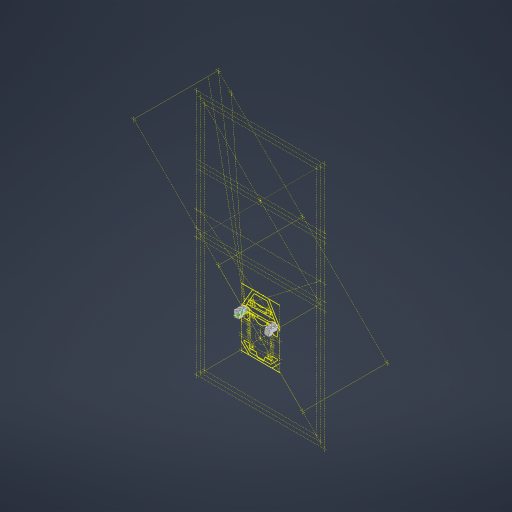
# Autodesk Inventor part: sensormount-2
Saved by Autodesk Inventor 2023.5 (Build 275446000, 446)
## iProperties
Created: 2025-01-19
Part Number: sensormount-2
Material: 一般
Document SubType Name: Modeling
Designer: IshiiLabHonda
Density: 1 g/cm^3
Appearance: 既定
Author: IshiiLabHonda
Autodesk Inventor part; units mm, degrees
ref_plane "YZ Plane" through (0, 0, 0) normal (1, 0, 0) x (0, 1, 0)
ref_plane "XZ Plane" through (0, 0, 0) normal (0, 1, 0) x (-1, 0, 0)
ref_plane "XY Plane" through (0, 0, 0) normal (0, 0, 1) x (1, 0, 0)
derived "chassis.ipt"
sketch "スケッチ1" plane through (0, 0, 0) normal (0, 0, 1) x (1, 0, 0)
  line L0 (-90, 90) -> (90, 90) construction
  line L1 (90, 90) -> (90, -90) construction
  line L2 (90, -90) -> (-90, -90) construction
  line L3 (-90, -90) -> (-90, 90) construction
  line L4 (-90, 90) -> (-90, 270) construction
  line L5 (-90, 270) -> (90, 270) construction
  line L6 (90, 270) -> (90, 90) construction
  line L7 (-90, 90) -> (90, -90) construction
  line L8 (90, 90) -> (-90, -90) construction
  line L9 (0, 0) -> (0, 10) construction
  line L10 (0, 0) -> (10, 0) construction
  line L11 (-90, 270) -> (90, 90) construction
  line L12 (-90, 90) -> (90, 270) construction
  line L13 (-96, 276) -> (96, 276) construction
  line L14 (96, 276) -> (96, -96) construction
  line L15 (96, -96) -> (-96, -96) construction
  line L16 (-96, -96) -> (-96, 276) construction
  line L17 (-84, 264) -> (84, 264) construction
  line L18 (84, 264) -> (84, -84) construction
  line L19 (84, -84) -> (-84, -84) construction
  line L20 (-84, -84) -> (-84, 264) construction
  line L21 (-96, 96) -> (96, 96) construction
  line L22 (-96, 84) -> (96, 84) construction
  line L23 (-63.6396, 63.6396) -> (63.6396, 190.9188) construction
  line L24 (63.6396, 190.9188) -> (190.9188, 63.6396) construction
  line L25 (190.9188, 63.6396) -> (63.6396, -63.6396) construction
  line L26 (63.6396, -63.6396) -> (-63.6396, 63.6396) construction
  line L27 (-190.9188, 190.9188) -> (-63.6396, 318.1981) construction
  line L28 (-63.6396, 318.1981) -> (63.6396, 190.9188) construction
  line L29 (-63.6396, 63.6396) -> (-190.9188, 190.9188) construction
  line L30 (-96, 120) -> (96, 120) construction
  line L31 (-96, 186) -> (96, 186) construction
  line L32 (-96, 174) -> (96, 174) construction
  line L33 (-96, 180) -> (96, 180) construction
  point P0 (-63.6396, 318.1981)
  point P1 (-90, 120)
  point P2 (90, 120)
  point P3 (0, 180)
sketch "スケッチ2" plane through (0, 0, 0) normal (0, 0, 1) x (1, 0, 0)
  line L0 (63.6396, 190.9188) -> (190.9188, 63.6396) construction
  line L1 (-63.6396, 318.1981) -> (63.6396, 190.9188) construction
  line L2 (-84, 264) -> (84, 264) construction
  line L3 (-90, 270) -> (90, 270) construction
  line L4 (90, 270) -> (90, 90) construction
  line L5 (-96, 276) -> (96, 276) construction
  line L6 (-90, 90) -> (90, 270) construction
  line L7 (-90, 270) -> (90, 90) construction
  line L8 (-63.6396, 63.6396) -> (63.6396, 190.9188) construction
  line L9 (-96, 120) -> (96, 120) construction
  line L10 (-90, 90) -> (90, 90) construction
  line L11 (-96, 96) -> (96, 96) construction
  line L12 (-96, 84) -> (96, 84) construction
  line L13 (90, -90) -> (-90, -90) construction
  line L14 (0, 0) -> (0, 10) construction
  line L15 (0, 0) -> (10, 0) construction
  line L16 (190.9188, 63.6396) -> (63.6396, -63.6396) construction
  line L17 (63.6396, -63.6396) -> (-63.6396, 63.6396) construction
  line L18 (84, -84) -> (-84, -84) construction
  line L19 (96, -96) -> (-96, -96) construction
  line L20 (-90, 90) -> (-90, 270) construction
  line L21 (-63.6396, 63.6396) -> (-190.9188, 190.9188) construction
  line L22 (-190.9188, 190.9188) -> (-63.6396, 318.1981) construction
  line L23 (96, 276) -> (96, -96) construction
  line L24 (-96, -96) -> (-96, 276) construction
  line L25 (84, 264) -> (84, -84) construction
  line L26 (-84, -84) -> (-84, 264) construction
  line L27 (90, 90) -> (90, -90) construction
  line L28 (-90, 90) -> (90, -90) construction
  line L29 (90, 90) -> (-90, -90) construction
  line L30 (-90, -90) -> (-90, 90) construction
  circle A0 centre (0, 0) radius 16 construction
  circle A1 centre (0, 0) radius 7.5 construction
  line L31 (20, 11.5) -> (28.75, 11.5) construction
  line L32 (28.75, 11.5) -> (28.75, -11.5) construction
  line L33 (28.75, -11.5) -> (20, -11.5) construction
  line L34 (20, -11.5) -> (20, 11.5) construction
  line L35 (20, 11.5) -> (18, 11.5) construction
  line L36 (18, 11.5) -> (18, -11.5) construction
  line L37 (18, -11.5) -> (20, -11.5) construction
  line L38 (18, 1.5) -> (17, 1.5) construction
  line L39 (17, -1.5) -> (18, -1.5) construction
  line L40 (-17, 26) -> (17, 26) construction
  line L41 (17, 26) -> (17, -20) construction
  line L42 (17, -20) -> (-17, -20) construction
  line L43 (-17, -20) -> (-17, 26) construction
  line L44 (-20, 11.5) -> (-18, 11.5) construction
  line L45 (-17, -1.5) -> (-18, -1.5) construction
  line L46 (-20, -11.5) -> (-20, 11.5) construction
  line L47 (-18, 11.5) -> (-18, -11.5) construction
  line L48 (-28.75, -11.5) -> (-20, -11.5) construction
  line L49 (-20, 11.5) -> (-28.75, 11.5) construction
  line L50 (-28.75, 11.5) -> (-28.75, -11.5) construction
  line L51 (-18, -11.5) -> (-20, -11.5) construction
  line L52 (-18, 1.5) -> (-17, 1.5) construction
  line L53 (-14.5, 26) -> (-14.5, -20) construction
  line L54 (14.5, 26) -> (14.5, -20) construction
  line L55 (-10.5, 26) -> (-10.5, 21) construction
  line L56 (-10.5, 21) -> (-14.5, 21) construction
  line L57 (-14.5, 26) -> (-10.5, 21) construction
  line L58 (-10.5, 26) -> (-14.5, 21) construction
  circle A2 centre (-12.5, 23.5) radius 1 construction
  line L59 (10.5, 26) -> (10.5, 21) construction
  line L60 (10.5, 21) -> (14.5, 21) construction
  line L61 (10.5, 26) -> (14.5, 21) construction
  line L62 (10.5, 21) -> (14.5, 26) construction
  circle A3 centre (12.5, 23.5) radius 1 construction
  line L63 (-14.5, -15) -> (-10.5, -15) construction
  line L64 (-10.5, -15) -> (-10.5, -20) construction
  line L65 (10.5, -20) -> (10.5, -15) construction
  line L66 (10.5, -15) -> (14.5, -15) construction
  line L67 (-14.5, -15) -> (-10.5, -20) construction
  line L68 (-10.5, -15) -> (-14.5, -20) construction
  circle A4 centre (-12.5, -17.5) radius 1 construction
  line L69 (10.5, -15) -> (14.5, -20) construction
  line L70 (14.5, -15) -> (10.5, -20) construction
  circle A5 centre (12.5, -17.5) radius 1 construction
  point P0 (90, 120)
  point P1 (-90, 120)
  point P2 (-63.6396, 318.1981)
  point P3 (-12.5, -17.5)
sketch "スケッチ3" plane through (0, 0, 0) normal (0, 0, 1) x (1, 0, 0)
  line L0 (63.6396, 190.9188) -> (190.9188, 63.6396) construction
  line L1 (-63.6396, 318.1981) -> (63.6396, 190.9188) construction
  line L2 (-84, 264) -> (84, 264) construction
  line L3 (-90, 270) -> (90, 270) construction
  line L4 (90, 270) -> (90, 90) construction
  line L5 (-96, 276) -> (96, 276) construction
  line L6 (-90, 90) -> (90, 270) construction
  line L7 (-90, 270) -> (90, 90) construction
  line L8 (-63.6396, 63.6396) -> (63.6396, 190.9188) construction
  line L9 (-96, 120) -> (96, 120) construction
  line L10 (-90, 90) -> (90, 90) construction
  line L11 (-96, 96) -> (96, 96) construction
  line L12 (-96, 84) -> (96, 84) construction
  line L13 (90, -90) -> (-90, -90) construction
  line L14 (0, 0) -> (0, 10) construction
  line L15 (0, 0) -> (10, 0) construction
  line L16 (190.9188, 63.6396) -> (63.6396, -63.6396) construction
  line L17 (63.6396, -63.6396) -> (-63.6396, 63.6396) construction
  line L18 (84, -84) -> (-84, -84) construction
  line L19 (96, -96) -> (-96, -96) construction
  line L20 (-90, 90) -> (-90, 270) construction
  line L21 (-63.6396, 63.6396) -> (-190.9188, 190.9188) construction
  line L22 (-190.9188, 190.9188) -> (-63.6396, 318.1981) construction
  line L23 (96, 276) -> (96, -96) construction
  line L24 (-96, -96) -> (-96, 276) construction
  line L25 (84, 264) -> (84, -84) construction
  line L26 (-84, -84) -> (-84, 264) construction
  line L27 (90, 90) -> (90, -90) construction
  line L28 (-90, 90) -> (90, -90) construction
  line L29 (90, 90) -> (-90, -90) construction
  line L30 (-90, -90) -> (-90, 90) construction
  line L31 (-18, 1.5) -> (-17, 1.5) construction
  line L32 (-17, -1.5) -> (-18, -1.5) construction
  line L33 (-20, 11.5) -> (-18, 11.5) construction
  line L34 (-28.75, 11.5) -> (-28.75, -11.5) construction
  line L35 (63.6396, -63.6396) -> (-63.6396, 63.6396) construction
  line L36 (84, -84) -> (-84, -84) construction
  line L37 (-90, -90) -> (-90, 90) construction
  line L38 (96, -96) -> (-96, -96) construction
  line L39 (-90, 90) -> (90, 90) construction
  line L40 (90, -90) -> (-90, -90) construction
  line L41 (90, 90) -> (-90, -90) construction
  line L42 (-90, 90) -> (90, -90) construction
  line L43 (90, 90) -> (90, -90) construction
  line L44 (-28.75, -11.5) -> (-20, -11.5) construction
  line L45 (-20, 11.5) -> (-28.75, 11.5) construction
  line L46 (-18, 11.5) -> (-18, -11.5) construction
  line L47 (-18, -11.5) -> (-20, -11.5) construction
  line L48 (0, 0) -> (0, 10) construction
  line L49 (0, 0) -> (10, 0) construction
  circle A0 centre (0, 0) radius 16 construction
  circle A1 centre (0, 0) radius 7.5 construction
  line L50 (-14.5, 26) -> (-14.5, -20) construction
  line L51 (-17, 26) -> (17, 26) construction
  line L52 (-17, -20) -> (-17, 26) construction
  line L53 (17, -20) -> (-17, -20) construction
  line L54 (-14.5, -15) -> (-10.5, -15) construction
  circle A2 centre (-12.5, -17.5) radius 1 construction
  line L55 (-10.5, -15) -> (-14.5, -20) construction
  line L56 (-14.5, -15) -> (-10.5, -20) construction
  line L57 (-63.6396, 318.1981) -> (63.6396, 190.9188) construction
  line L58 (-84, 264) -> (84, 264) construction
  line L59 (-90, 270) -> (90, 270) construction
  line L60 (90, 270) -> (90, 90) construction
  line L61 (-96, 276) -> (96, 276) construction
  line L62 (-90, 90) -> (90, 270) construction
  line L63 (-90, 270) -> (90, 90) construction
  line L64 (-63.6396, 63.6396) -> (63.6396, 190.9188) construction
  line L65 (-96, 120) -> (96, 120) construction
  line L66 (-96, 96) -> (96, 96) construction
  line L67 (-96, 84) -> (96, 84) construction
  line L68 (84, 264) -> (84, -84) construction
  line L69 (96, 276) -> (96, -96) construction
  line L70 (-96, -96) -> (-96, 276) construction
  line L71 (-84, -84) -> (-84, 264) construction
  line L72 (-63.6396, 63.6396) -> (-190.9188, 190.9188) construction
  line L73 (-90, 90) -> (-90, 270) construction
  line L74 (-190.9188, 190.9188) -> (-63.6396, 318.1981) construction
  line L75 (-20, -11.5) -> (-20, 11.5) construction
  line L76 (10.5, -15) -> (14.5, -15) construction
  line L77 (10.5, -20) -> (10.5, -15) construction
  circle A3 centre (12.5, -17.5) radius 1 construction
  line L78 (10.5, -15) -> (14.5, -20) construction
  line L79 (14.5, -15) -> (10.5, -20) construction
  line L80 (-10.5, -15) -> (-10.5, -20) construction
  line L81 (63.6396, 190.9188) -> (190.9188, 63.6396) construction
  line L82 (190.9188, 63.6396) -> (63.6396, -63.6396) construction
  line L83 (20, 11.5) -> (28.75, 11.5) construction
  line L84 (28.75, 11.5) -> (28.75, -11.5) construction
  line L85 (17, -1.5) -> (18, -1.5) construction
  line L86 (18, -11.5) -> (20, -11.5) construction
  line L87 (28.75, -11.5) -> (20, -11.5) construction
  line L88 (14.5, 26) -> (14.5, -20) construction
  line L89 (17, 26) -> (17, -20) construction
  line L90 (18, 11.5) -> (18, -11.5) construction
  line L91 (20, -11.5) -> (20, 11.5) construction
  line L92 (20, 11.5) -> (18, 11.5) construction
  line L93 (18, 1.5) -> (17, 1.5) construction
  line L94 (-10.5, 26) -> (-10.5, 21) construction
  line L95 (10.5, 21) -> (14.5, 21) construction
  circle A4 centre (12.5, 23.5) radius 1 construction
  line L96 (10.5, 26) -> (14.5, 21) construction
  line L97 (10.5, 21) -> (14.5, 26) construction
  line L98 (10.5, 26) -> (10.5, 21) construction
  line L99 (-10.5, 21) -> (-14.5, 21) construction
  circle A5 centre (-12.5, 23.5) radius 1 construction
  line L100 (-14.5, 26) -> (-10.5, 21) construction
  line L101 (-10.5, 26) -> (-14.5, 21) construction
  line L102 (29.25, 58) -> (29.25, -32) construction
  line L103 (29.25, -32) -> (-29.25, -32) construction
  line L104 (-29.25, -32) -> (-29.25, 58) construction
  line L105 (-29.25, 8.5) -> (-17, 8.5) construction
  line L106 (-17, 8.5) -> (-17, -8.5) construction
  line L107 (-17, -8.5) -> (-29.25, -8.5) construction
  line L108 (29.25, 8.5) -> (17, 8.5) construction
  line L109 (17, 8.5) -> (17, -8.5) construction
  line L110 (17, -8.5) -> (29.25, -8.5) construction
  line L111 (-20.1078, 31.6026) -> (-18.8984, 22.9366) construction
  line L112 (7.9335, 41.7018) -> (10.9773, 45.6686) construction
  line L113 (6.7297, 41.365) -> (10.991, 46.9185) construction
  line L114 (11.8865, 37.4081) -> (6.7297, 41.365) construction
  line L115 (10.991, 46.9185) -> (11.8865, 37.4081) construction
  line L116 (11.9003, 38.658) -> (10.9773, 45.6686) construction
  line L117 (11.9003, 38.658) -> (7.9335, 41.7018) construction
  line L118 (11.8865, 37.4081) -> (14.2666, 35.5818) construction
  line L119 (10.9773, 45.6686) -> (14.9441, 42.6248) construction
  line L120 (7.9335, 41.7018) -> (14.9441, 42.6248) construction
  line L121 (14.9441, 42.6248) -> (11.9003, 38.658) construction
  line L122 (6.7297, 41.365) -> (16.1478, 42.9616) construction
  line L123 (10.991, 46.9185) -> (16.1478, 42.9616) construction
  line L124 (16.1478, 42.9616) -> (11.8865, 37.4081) construction
  line L125 (14.2666, 35.5818) -> (18.5279, 41.1353) construction
  line L126 (18.5279, 41.1353) -> (16.1478, 42.9616) construction
  line L127 (-20.9946, 30.7216) -> (-20.3034, 25.7696) construction
  line L128 (-25.9466, 30.0304) -> (-20.3034, 25.7696) construction
  line L129 (-25.2554, 25.0784) -> (-20.9946, 30.7216) construction
  line L130 (-27.0406, 30.635) -> (-20.1078, 31.6026) construction
  line L131 (-25.2554, 25.0784) -> (-25.9466, 30.0304) construction
  line L132 (-18.8984, 22.9366) -> (-25.8312, 21.969) construction
  line L133 (-25.8312, 21.969) -> (-27.0406, 30.635) construction
  line L134 (-63.6396, 318.1981) -> (-23.125, 27.9) construction
  line L135 (11.4388, 42.1633) -> (-90, 120) construction
  line L136 (-23.125, 27.9) -> (-78.8228, 303.0149) construction
  line L137 (-23.125, 27.9) -> (-44.1788, 298.7372) construction
  line L138 (-11.4388, 42.1633) -> (90, 120) construction
  line L139 (-10.9773, 45.6686) -> (-7.9335, 41.7018) construction
  line L140 (-10.991, 46.9185) -> (-6.7297, 41.365) construction
  line L141 (-16.1478, 42.9616) -> (-10.991, 46.9185) construction
  line L142 (-6.7297, 41.365) -> (-16.1478, 42.9616) construction
  line L143 (-14.9441, 42.6248) -> (-7.9335, 41.7018) construction
  line L144 (-14.9441, 42.6248) -> (-10.9773, 45.6686) construction
  line L145 (-16.1478, 42.9616) -> (-18.5279, 41.1353) construction
  line L146 (-7.9335, 41.7018) -> (-11.9003, 38.658) construction
  line L147 (-10.9773, 45.6686) -> (-11.9003, 38.658) construction
  line L148 (-10.991, 46.9185) -> (-11.8865, 37.4081) construction
  line L149 (-6.7297, 41.365) -> (-11.8865, 37.4081) construction
  line L150 (-11.8865, 37.4081) -> (-16.1478, 42.9616) construction
  line L151 (-18.5279, 41.1353) -> (-14.2666, 35.5818) construction
  line L152 (-14.2666, 35.5818) -> (-11.8865, 37.4081) construction
  line L153 (-11.9003, 38.658) -> (-14.9441, 42.6248) construction
  circle A6 centre (-8.395, 38.1965) radius 0.625 construction
  circle A7 centre (-8.395, 38.1965) radius 0.8 construction
  circle A8 centre (-8.395, 38.1965) radius 1.5 construction
  circle A9 centre (-15.2072, 39.2717) radius 1.5 construction
  circle A10 centre (-15.2072, 39.2717) radius 0.8 construction
  circle A11 centre (-15.2072, 39.2717) radius 0.625 construction
  line L154 (-20.3034, 25.7696) -> (-25.2554, 25.0784) construction
  line L155 (-26.1422, 24.1974) -> (-19.2094, 25.165) construction
  line L156 (-25.601, 27.5544) -> (-20.649, 28.2456) construction
  line L157 (-22.3648, 22.4528) -> (-22.7794, 25.424) construction
  circle A12 centre (-18.173, 28.5911) radius 0.625 construction
  circle A13 centre (-18.173, 28.5911) radius 0.8 construction
  circle A14 centre (-18.173, 28.5911) radius 1.5 construction
  circle A15 centre (-27.1405, 25.3286) radius 0.625 construction
  circle A16 centre (-27.1405, 25.3286) radius 0.8 construction
  line L158 (-25.9466, 30.0304) -> (-20.9946, 30.7216) construction
  circle A17 centre (18.173, 28.5911) radius 0.625 construction
  circle A18 centre (18.173, 28.5911) radius 0.8 construction
  circle A19 centre (18.173, 28.5911) radius 1.5
  circle A20 centre (27.1405, 25.3286) radius 0.625
  circle A21 centre (27.1405, 25.3286) radius 0.8 construction
  circle A22 centre (27.1405, 25.3286) radius 1.5
  circle A23 centre (15.2072, 39.2717) radius 1.5 construction
  circle A24 centre (15.2072, 39.2717) radius 0.625 construction
  circle A25 centre (15.2072, 39.2717) radius 0.8
  circle A26 centre (8.395, 38.1965) radius 1.5 construction
  circle A27 centre (8.395, 38.1965) radius 0.8
  circle A28 centre (8.395, 38.1965) radius 0.625 construction
  line L159 (-29.25, -32) -> (29.25, -32)
  line L160 (-29.25, 58) -> (29.25, 58)
  line L161 (-11.4388, 42.1633) -> (-8.395, 38.1965) construction
  line L162 (-29.25, 28.2016) -> (-12.0459, 58)
  line L163 (-29.25, -17.6878) -> (-14.9378, -32)
  line L164 (29.25, 28.2016) -> (12.0459, 58)
  line L165 (29.25, -17.6878) -> (14.9378, -32)
  line L166 (-9.7365, 54) -> (9.7365, 54)
  line L167 (9.7365, 54) -> (25.25, 27.1298)
  line L168 (25.25, 27.1298) -> (25.25, 14.5)
  line L169 (25.25, 14.5) -> (17, 14.5)
  line L170 (3.695, 18.0905) -> (-3.695, 18.0905)
  line L171 (-17, 14.5) -> (-25.25, 14.5)
  line L172 (-25.25, 14.5) -> (-25.25, 27.1298)
  line L173 (-25.25, 27.1298) -> (-9.7365, 54)
  line L174 (18.8984, 22.9366) -> (25.8312, 21.969) construction
  line L175 (25.8312, 21.969) -> (27.0406, 30.635) construction
  line L176 (20.1078, 31.6026) -> (18.8984, 22.9366) construction
  line L177 (20.3034, 25.7696) -> (25.2554, 25.0784) construction
  line L178 (26.1422, 24.1974) -> (19.2094, 25.165) construction
  line L179 (25.9466, 30.0304) -> (20.3034, 25.7696) construction
  line L180 (25.2554, 25.0784) -> (20.9946, 30.7216) construction
  line L181 (20.9946, 30.7216) -> (20.3034, 25.7696) construction
  line L182 (25.9466, 30.0304) -> (20.9946, 30.7216) construction
  line L183 (25.2554, 25.0784) -> (25.9466, 30.0304) construction
  line L184 (27.0406, 30.635) -> (20.1078, 31.6026) construction
  line L185 (-9.7365, 22.9366) -> (-9.7365, 26)
  line L186 (9.7365, 22.9366) -> (9.7365, 26)
  line L187 (9.7365, 26) -> (17, 26)
  line L188 (17, 26) -> (17, 14.5)
  line L189 (-9.7365, 26) -> (-17, 26)
  line L190 (-17, 26) -> (-17, 14.5)
  line L191 (-9.7365, 22.9366) -> (-3.695, 18.0905)
  line L192 (9.7365, 22.9366) -> (3.695, 18.0905)
  line L193 (-17, -14.5) -> (-25.25, -14.5)
  line L194 (-25.25, -14.5) -> (-25.25, -16.0309)
  line L195 (-25.25, -16.0309) -> (-13.2809, -28)
  line L196 (-13.2809, -28) -> (13.2809, -28)
  line L197 (13.2809, -28) -> (25.25, -16.0309)
  line L198 (25.25, -16.0309) -> (25.25, -14.5)
  line L199 (25.25, -14.5) -> (17, -14.5)
  line L200 (17, -14.5) -> (17, -20.8804)
  line L201 (17, -20.8804) -> (6.6466, -20.8804)
  line L202 (6.6466, -20.8804) -> (4.7017, -18.0332)
  line L203 (4.7017, -18.0332) -> (-4.7017, -18.0332)
  line L204 (-4.7017, -18.0332) -> (-6.6466, -20.8804)
  line L205 (-6.6466, -20.8804) -> (-17, -20.8804)
  line L206 (-17, -20.8804) -> (-17, -14.5)
  line L207 (-16.1661, 42.8636) -> (16.1661, 42.8636)
  line L208 (-20.6579, 35.0836) -> (20.6579, 35.0836)
  line L209 (-22.045, 32.6811) -> (-12.2942, 28.5594)
  line L210 (-12.2942, 28.5594) -> (12.2942, 28.5594)
  line L211 (12.2942, 28.5594) -> (22.045, 32.6811)
  line L212 (-25.25, 25.1515) -> (25.25, 25.1515)
  circle A29 centre (-27.1405, 25.3286) radius 1.5 construction
  line L213 (-7.5571, 35.0836) -> (-5.0762, 37.1727)
  line L214 (-5.0762, 37.1727) -> (5.0762, 37.1727)
  line L215 (5.0762, 37.1727) -> (7.5571, 35.0836)
  line L216 (0, 41.1322) -> (6.2476, 42.8636)
  line L217 (-6.2476, 42.8636) -> (0, 41.1322)
  line L218 (-17, 18.9574) -> (-20.6579, 14.5)
  line L219 (17, 18.9574) -> (20.6579, 14.5)
  point P0 (16.5079, 42.2717)
  point P1 (-4.3925, 58)
  point P2 (4.5158, 58)
sketch "スケッチ4" plane through (0, 0, 0) normal (0, 0, 1) x (1, 0, 0)
  line L0 (-90, 90) -> (90, 90) construction
  line L1 (90, 90) -> (90, -90) construction
  line L2 (90, -90) -> (-90, -90) construction
  line L3 (-90, -90) -> (-90, 90) construction
  line L4 (0, 0) -> (0, 10) construction
  line L5 (0, 0) -> (10, 0) construction
  line L6 (63.6396, -63.6396) -> (-63.6396, 63.6396) construction
  line L7 (-90, 90) -> (90, -90) construction
  line L8 (90, 90) -> (-90, -90) construction
  line L9 (84, -84) -> (-84, -84) construction
  line L10 (96, -96) -> (-96, -96) construction
  line L11 (-90, 270) -> (90, 270) construction
  line L12 (-84, 264) -> (84, 264) construction
  line L13 (-63.6396, 318.1981) -> (63.6396, 190.9188) construction
  line L14 (-96, 276) -> (96, 276) construction
  line L15 (-90, 90) -> (-90, 270) construction
  line L16 (-96, 84) -> (96, 84) construction
  line L17 (-96, 96) -> (96, 96) construction
  line L18 (-96, 120) -> (96, 120) construction
  line L19 (96, 276) -> (96, -96) construction
  line L20 (-96, -96) -> (-96, 276) construction
  line L21 (-84, -84) -> (-84, 264) construction
  line L22 (84, 264) -> (84, -84) construction
  line L23 (-63.6396, 63.6396) -> (63.6396, 190.9188) construction
  line L24 (-96, 180) -> (96, 180) construction
  line L25 (-96, 186) -> (96, 186) construction
  line L26 (-90, 270) -> (90, 90) construction
  line L27 (90, 270) -> (90, 90) construction
  line L28 (-90, 90) -> (90, 270) construction
  line L29 (-96, 174) -> (96, 174) construction
  line L30 (-190.9188, 190.9188) -> (-63.6396, 318.1981) construction
  line L31 (-63.6396, 63.6396) -> (-190.9188, 190.9188) construction
  line L32 (63.6396, 190.9188) -> (190.9188, 63.6396) construction
  line L33 (190.9188, 63.6396) -> (63.6396, -63.6396) construction
  line L34 (-63.6396, 63.6396) -> (-190.9188, 190.9188) construction
  line L35 (-90, 90) -> (-90, 270) construction
  line L36 (-190.9188, 190.9188) -> (-63.6396, 318.1981) construction
  line L37 (0, 0) -> (0, 10) construction
  line L38 (-10.5, 21) -> (-14.5, 21) construction
  circle A0 centre (0, 0) radius 7.5 construction
  line L39 (-10.5, 26) -> (-14.5, 21) construction
  line L40 (-14.5, 26) -> (-10.5, 21) construction
  line L41 (0, 0) -> (10, 0) construction
  line L42 (-17, -20) -> (-17, 26) construction
  circle A1 centre (0, 0) radius 16 construction
  line L43 (-14.5, 26) -> (-14.5, -20) construction
  line L44 (17, -20) -> (-17, -20) construction
  line L45 (-17, 26) -> (17, 26) construction
  line L46 (14.5, 26) -> (14.5, -20) construction
  line L47 (17, 26) -> (17, -20) construction
  line L48 (18, 11.5) -> (18, -11.5) construction
  line L49 (20, -11.5) -> (20, 11.5) construction
  line L50 (-18, 11.5) -> (-18, -11.5) construction
  line L51 (-20, -11.5) -> (-20, 11.5) construction
  line L52 (-17, -1.5) -> (-18, -1.5) construction
  line L53 (-20, 11.5) -> (-18, 11.5) construction
  line L54 (-18, 1.5) -> (-17, 1.5) construction
  line L55 (190.9188, 63.6396) -> (63.6396, -63.6396) construction
  line L56 (20, 11.5) -> (28.75, 11.5) construction
  line L57 (28.75, 11.5) -> (28.75, -11.5) construction
  line L58 (17, -1.5) -> (18, -1.5) construction
  line L59 (18, 1.5) -> (17, 1.5) construction
  line L60 (20, 11.5) -> (18, 11.5) construction
  circle A2 centre (-12.5, 23.5) radius 1 construction
  line L61 (-18, -11.5) -> (-20, -11.5) construction
  line L62 (63.6396, 190.9188) -> (190.9188, 63.6396) construction
  line L63 (-63.6396, 318.1981) -> (63.6396, 190.9188) construction
  line L64 (-84, 264) -> (84, 264) construction
  line L65 (-90, 270) -> (90, 270) construction
  line L66 (90, 270) -> (90, 90) construction
  line L67 (-96, 276) -> (96, 276) construction
  line L68 (-20, 11.5) -> (-28.75, 11.5) construction
  line L69 (-63.6396, 63.6396) -> (63.6396, 190.9188) construction
  line L70 (-28.75, 11.5) -> (-28.75, -11.5) construction
  line L71 (-28.75, -11.5) -> (-20, -11.5) construction
  line L72 (-90, 90) -> (90, 270) construction
  line L73 (-90, 270) -> (90, 90) construction
  line L74 (-90, 90) -> (90, 90) construction
  line L75 (-96, 120) -> (96, 120) construction
  line L76 (-96, 96) -> (96, 96) construction
  line L77 (-96, 84) -> (96, 84) construction
  line L78 (-84, -84) -> (-84, 264) construction
  line L79 (-96, -96) -> (-96, 276) construction
  line L80 (84, 264) -> (84, -84) construction
  line L81 (96, 276) -> (96, -96) construction
  line L82 (-90, -90) -> (-90, 90) construction
  line L83 (63.6396, -63.6396) -> (-63.6396, 63.6396) construction
  line L84 (84, -84) -> (-84, -84) construction
  line L85 (90, -90) -> (-90, -90) construction
  line L86 (90, 90) -> (90, -90) construction
  line L87 (-90, 90) -> (90, -90) construction
  line L88 (96, -96) -> (-96, -96) construction
  line L89 (90, 90) -> (-90, -90) construction
  line L90 (10.5, 26) -> (10.5, 21) construction
  line L91 (10.5, 21) -> (14.5, 21) construction
  circle A3 centre (12.5, 23.5) radius 1 construction
  line L92 (10.5, 21) -> (14.5, 26) construction
  line L93 (10.5, 26) -> (14.5, 21) construction
  line L94 (-10.5, 26) -> (-10.5, 21) construction
  line L95 (28.75, -11.5) -> (20, -11.5) construction
  line L96 (18, -11.5) -> (20, -11.5) construction
  circle A4 centre (12.5, -17.5) radius 1 construction
  line L97 (-14.5, -15) -> (-10.5, -15) construction
  circle A5 centre (-12.5, -17.5) radius 1 construction
  line L98 (-14.5, -15) -> (-10.5, -20) construction
  line L99 (-10.5, -15) -> (-14.5, -20) construction
  line L100 (-10.5, -15) -> (-10.5, -20) construction
  line L101 (10.5, -15) -> (14.5, -15) construction
  line L102 (10.5, -20) -> (10.5, -15) construction
  line L103 (10.5, -15) -> (14.5, -20) construction
  line L104 (14.5, -15) -> (10.5, -20) construction
  line L105 (-96, 96) -> (96, 96) construction
  line L106 (-96, 84) -> (96, 84) construction
  line L107 (-96, 84) -> (96, 84) construction
  line L108 (96, -96) -> (-96, -96) construction
  line L109 (96, -96) -> (-96, -96) construction
  line L110 (-96, 96) -> (96, 96) construction
  circle A6 centre (-8.395, 38.1965) radius 1.5 construction
  line L111 (-20, 11.5) -> (-28.75, 11.5) construction
  line L112 (-20, 11.5) -> (-18, 11.5) construction
  line L113 (-18, 1.5) -> (-17, 1.5) construction
  line L114 (-28.75, 11.5) -> (-28.75, -11.5) construction
  line L115 (-28.75, -11.5) -> (-20, -11.5) construction
  line L116 (63.6396, -63.6396) -> (-63.6396, 63.6396) construction
  line L117 (63.6396, -63.6396) -> (-63.6396, 63.6396) construction
  line L118 (-90, 90) -> (90, 90) construction
  line L119 (-90, 90) -> (90, 90) construction
  line L120 (-90, -90) -> (-90, 90) construction
  line L121 (-90, -90) -> (-90, 90) construction
  line L122 (90, 90) -> (90, -90) construction
  line L123 (90, 90) -> (90, -90) construction
  line L124 (90, 90) -> (-90, -90) construction
  line L125 (90, 90) -> (-90, -90) construction
  line L126 (-90, 90) -> (90, -90) construction
  line L127 (-90, 90) -> (90, -90) construction
  line L128 (84, -84) -> (-84, -84) construction
  line L129 (90, -90) -> (-90, -90) construction
  line L130 (90, -90) -> (-90, -90) construction
  line L131 (84, -84) -> (-84, -84) construction
  line L132 (-84, 264) -> (84, 264) construction
  line L133 (-90, 90) -> (90, 270) construction
  line L134 (-90, 90) -> (90, 270) construction
  line L135 (-84, 264) -> (84, 264) construction
  line L136 (-14.9441, 42.6248) -> (-7.9335, 41.7018) construction
  line L137 (-17, -1.5) -> (-18, -1.5) construction
  circle A7 centre (-8.395, 38.1965) radius 0.8 construction
  line L138 (-14.9441, 42.6248) -> (-10.9773, 45.6686) construction
  circle A8 centre (-15.2072, 39.2717) radius 0.625 construction
  line L139 (-17, -20) -> (-17, 26) construction
  circle A9 centre (-15.2072, 39.2717) radius 0.8 construction
  line L140 (-14.2666, 35.5818) -> (-11.8865, 37.4081) construction
  circle A10 centre (-15.2072, 39.2717) radius 1.5 construction
  line L141 (-18.5279, 41.1353) -> (-14.2666, 35.5818) construction
  line L142 (-16.1478, 42.9616) -> (-18.5279, 41.1353) construction
  line L143 (-11.8865, 37.4081) -> (-16.1478, 42.9616) construction
  line L144 (-11.9003, 38.658) -> (-14.9441, 42.6248) construction
  line L145 (-25.9466, 30.0304) -> (-20.9946, 30.7216) construction
  line L146 (-20.9946, 30.7216) -> (-20.3034, 25.7696) construction
  line L147 (-22.3648, 22.4528) -> (-22.7794, 25.424) construction
  line L148 (-25.2554, 25.0784) -> (-20.9946, 30.7216) construction
  line L149 (-25.9466, 30.0304) -> (-20.3034, 25.7696) construction
  line L150 (-20.3034, 25.7696) -> (-25.2554, 25.0784) construction
  line L151 (-25.2554, 25.0784) -> (-25.9466, 30.0304) construction
  line L152 (-25.601, 27.5544) -> (-20.649, 28.2456) construction
  line L153 (0, 0) -> (0, 10) construction
  line L154 (0, 0) -> (10, 0) construction
  line L155 (-18, 11.5) -> (-18, -11.5) construction
  line L156 (-18, -11.5) -> (-20, -11.5) construction
  line L157 (0, 0) -> (0, 10) construction
  line L158 (0, 0) -> (10, 0) construction
  circle A11 centre (0, 0) radius 16 construction
  circle A12 centre (0, 0) radius 7.5 construction
  line L159 (-17, 26) -> (17, 26) construction
  line L160 (17, -20) -> (-17, -20) construction
  line L161 (-14.5, 26) -> (-14.5, -20) construction
  line L162 (-27.0406, 30.635) -> (-20.1078, 31.6026) projected
  line L163 (-10.5, 21) -> (-14.5, 21) construction
  line L164 (-10.5, 26) -> (-10.5, 21) construction
  circle A13 centre (-12.5, 23.5) radius 1 construction
  line L165 (-14.5, 26) -> (-10.5, 21) construction
  line L166 (-29.25, 8.5) -> (-17, 8.5) construction
  line L167 (-10.5, 26) -> (-14.5, 21) construction
  line L168 (11.8865, 37.4081) -> (14.2666, 35.5818) construction
  line L169 (14.2666, 35.5818) -> (18.5279, 41.1353) construction
  line L170 (-20.1078, 31.6026) -> (-18.8984, 22.9366) projected
  line L171 (-18.8984, 22.9366) -> (-25.8312, 21.969) construction
  circle A14 centre (-27.1405, 25.3286) radius 0.625 projected
  circle A15 centre (-27.1405, 25.3286) radius 0.8 construction
  line L172 (-26.1422, 24.1974) -> (-19.2094, 25.165) projected
  circle A16 centre (-18.173, 28.5911) radius 0.625 projected
  circle A17 centre (-18.173, 28.5911) radius 0.8 construction
  circle A18 centre (-18.173, 28.5911) radius 1.5 projected
  line L173 (-25.8312, 21.969) -> (-27.0406, 30.635) projected
  line L174 (-6.7297, 41.365) -> (-16.1478, 42.9616) construction
  line L175 (-16.1478, 42.9616) -> (-10.991, 46.9185) construction
  line L176 (-20, -11.5) -> (-20, 11.5) construction
  line L177 (10.5, -15) -> (14.5, -15) construction
  line L178 (-17, 8.5) -> (-17, -8.5) construction
  line L179 (-17, -8.5) -> (-29.25, -8.5) construction
  line L180 (-10.5, -15) -> (-10.5, -20) construction
  line L181 (20, 11.5) -> (18, 11.5) construction
  line L182 (18, 1.5) -> (17, 1.5) construction
  line L183 (17, -1.5) -> (18, -1.5) construction
  line L184 (18, 11.5) -> (18, -11.5) construction
  line L185 (18, -11.5) -> (20, -11.5) construction
  line L186 (10.5, -20) -> (10.5, -15) construction
  circle A19 centre (12.5, -17.5) radius 1 construction
  line L187 (10.5, -15) -> (14.5, -20) construction
  line L188 (14.5, -15) -> (10.5, -20) construction
  line L189 (-29.25, -32) -> (-29.25, 58) construction
  line L190 (29.25, -32) -> (-29.25, -32) construction
  line L191 (14.5, 26) -> (14.5, -20) construction
  line L192 (17, 26) -> (17, -20) construction
  line L193 (28.75, 11.5) -> (28.75, -11.5) construction
  line L194 (28.75, -11.5) -> (20, -11.5) construction
  line L195 (17, 8.5) -> (17, -8.5) construction
  line L196 (-63.6396, 63.6396) -> (63.6396, 190.9188) construction
  line L197 (-63.6396, 63.6396) -> (63.6396, 190.9188) construction
  line L198 (-63.6396, 318.1981) -> (63.6396, 190.9188) construction
  line L199 (-90, 270) -> (90, 270) construction
  line L200 (90, 270) -> (90, 90) construction
  line L201 (-96, 120) -> (96, 120) construction
  line L202 (-96, 120) -> (96, 120) construction
  line L203 (11.4388, 42.1633) -> (-90, 120) construction
  line L204 (-96, -96) -> (-96, 276) construction
  line L205 (-96, -96) -> (-96, 276) construction
  line L206 (96, 276) -> (96, -96) construction
  line L207 (96, 276) -> (96, -96) construction
  line L208 (-84, -84) -> (-84, 264) construction
  line L209 (-84, -84) -> (-84, 264) construction
  line L210 (84, 264) -> (84, -84) construction
  line L211 (84, 264) -> (84, -84) construction
  line L212 (-90, 90) -> (-90, 270) construction
  line L213 (-90, 90) -> (-90, 270) construction
  line L214 (-90, 270) -> (90, 90) construction
  line L215 (-90, 270) -> (90, 90) construction
  line L216 (90, 270) -> (90, 90) construction
  line L217 (-23.125, 27.9) -> (-44.1788, 298.7372) construction
  line L218 (-23.125, 27.9) -> (-78.8228, 303.0149) construction
  line L219 (-63.6396, 318.1981) -> (-23.125, 27.9) construction
  line L220 (-90, 270) -> (90, 270) construction
  line L221 (-96, 276) -> (96, 276) construction
  line L222 (-96, 276) -> (96, 276) construction
  line L223 (-63.6396, 318.1981) -> (63.6396, 190.9188) construction
  line L224 (-63.6396, 63.6396) -> (-190.9188, 190.9188) construction
  line L225 (-63.6396, 63.6396) -> (-190.9188, 190.9188) construction
  line L226 (-190.9188, 190.9188) -> (-63.6396, 318.1981) construction
  line L227 (-190.9188, 190.9188) -> (-63.6396, 318.1981) construction
  line L228 (-14.5, -15) -> (-10.5, -15) construction
  circle A20 centre (-12.5, -17.5) radius 1 construction
  line L229 (-14.5, -15) -> (-10.5, -20) construction
  line L230 (-10.5, -15) -> (-14.5, -20) construction
  line L231 (10.9773, 45.6686) -> (14.9441, 42.6248) construction
  line L232 (7.9335, 41.7018) -> (14.9441, 42.6248) construction
  line L233 (-10.9773, 45.6686) -> (-7.9335, 41.7018) construction
  line L234 (6.7297, 41.365) -> (16.1478, 42.9616) construction
  line L235 (-10.991, 46.9185) -> (-6.7297, 41.365) construction
  line L236 (18.5279, 41.1353) -> (16.1478, 42.9616) construction
  line L237 (11.9003, 38.658) -> (10.9773, 45.6686) construction
  line L238 (11.9003, 38.658) -> (7.9335, 41.7018) construction
  line L239 (14.9441, 42.6248) -> (11.9003, 38.658) construction
  line L240 (16.1478, 42.9616) -> (11.8865, 37.4081) construction
  line L241 (10.991, 46.9185) -> (11.8865, 37.4081) construction
  line L242 (11.8865, 37.4081) -> (6.7297, 41.365) construction
  circle A21 centre (-8.395, 38.1965) radius 0.625 construction
  line L243 (-7.9335, 41.7018) -> (-11.9003, 38.658) construction
  line L244 (-10.9773, 45.6686) -> (-11.9003, 38.658) construction
  line L245 (-10.991, 46.9185) -> (-11.8865, 37.4081) construction
  line L246 (-6.7297, 41.365) -> (-11.8865, 37.4081) construction
  line L247 (7.9335, 41.7018) -> (10.9773, 45.6686) construction
  line L248 (6.7297, 41.365) -> (10.991, 46.9185) construction
  line L249 (20, -11.5) -> (20, 11.5) construction
  line L250 (20, 11.5) -> (28.75, 11.5) construction
  line L251 (10.5, 21) -> (14.5, 21) construction
  line L252 (10.5, 26) -> (14.5, 21) construction
  line L253 (10.5, 21) -> (14.5, 26) construction
  line L254 (10.5, 26) -> (10.5, 21) construction
  line L255 (17, -8.5) -> (29.25, -8.5) construction
  circle A22 centre (12.5, 23.5) radius 1 construction
  line L256 (-11.4388, 42.1633) -> (90, 120) construction
  line L257 (63.6396, 190.9188) -> (190.9188, 63.6396) construction
  line L258 (63.6396, 190.9188) -> (190.9188, 63.6396) construction
  line L259 (10.991, 46.9185) -> (16.1478, 42.9616) construction
  line L260 (190.9188, 63.6396) -> (63.6396, -63.6396) construction
  line L261 (190.9188, 63.6396) -> (63.6396, -63.6396) construction
  line L262 (29.25, 8.5) -> (17, 8.5) construction
  circle A23 centre (8.395, 38.1965) radius 0.625 construction
  circle A24 centre (8.395, 38.1965) radius 0.8 projected
  circle A25 centre (27.1405, 25.3286) radius 0.625 projected
  circle A26 centre (27.1405, 25.3286) radius 0.8 construction
  circle A27 centre (15.2072, 39.2717) radius 0.625 construction
  circle A28 centre (15.2072, 39.2717) radius 0.8 projected
  circle A29 centre (15.2072, 39.2717) radius 1.5 construction
  circle A30 centre (18.173, 28.5911) radius 0.625 projected
  circle A31 centre (18.173, 28.5911) radius 0.8 construction
  circle A32 centre (18.173, 28.5911) radius 1.5 projected
  circle A33 centre (27.1405, 25.3286) radius 1.5 projected
  circle A34 centre (-27.1405, 25.3286) radius 1.5 projected
  point P0 (0, 180)
  point P1 (-12.5, -17.5)
  point P2 (8.395, 38.1965)
  constraints: 67 other
extrude "押し出し1" add sketch "スケッチ4" along normal blind 13.5 contours L162 L170 L172 L173 A34 | A34 L173 picked at (-26.0311, 25.3785)
ref_plane "作業平面1" through (-19.2094, 25.165, 0) normal (0.1382225, -0.9904012, 0) x (0.9904012, 0.1382225, 0)
sketch "スケッチ5" plane through (-19.2094, 25.165, 0) normal (0.1382225, -0.9904012, 0) x (0.9904012, 0.1382225, 0)
  line L0 (-7, 0) -> (0, 0) projected
  line L1 (0, 0) -> (0, 13.5) projected
  line L2 (-7, 13.5) -> (0, 13.5) projected
  line L3 (-7, 0) -> (-7, 13.5) projected
  line L4 (-7, 12.5) -> (0, 12.5)
  line L5 (-7, 7.5) -> (0, 7.5)
  line L6 (-7, 6.5) -> (0, 6.5)
  line L7 (-7, 1.5) -> (0, 1.5)
  line L8 (-7, 13.5) -> (0, 13.5) projected
  line L9 (-7, 0) -> (0, 0) projected
  line L10 (-7, 13.5) -> (0, 0) construction
  line L11 (0, 13.5) -> (-7, 0) construction
  line L12 (-3.5, 13.5) -> (-3.5, 0) construction
  line L13 (-7, 1.5) -> (0, 6.5) construction
  circle A0 centre (-3.5, 4) radius 2.5
  line L14 (-7, 12.5) -> (0, 7.5) construction
  line L15 (-7, 7.5) -> (0, 12.5) construction
  circle A1 centre (-3.5, 10) radius 2.5
  line L16 (-7, 7) -> (0, 7)
  point P0 (15.5466, 0)
  point P1 (-3.5, 6.75)
  point P2 (-3.5, 6.75)
  dimension "d4" = 1.5
  dimension "d5" = 1
  dimension "d6" = 1
  dimension "d7" = 5
  dimension "d8" = 5
  constraints: 22 end point, 10 point on line, 7 midpoint, 4 parallel, 2 centre point, 1 perpendicular, 1 tangent, 1 other
  measures "d4" distance between parallel lines of L0 L7
  measures "d5" distance between parallel lines of L5 L6
  measures "d6" distance between parallel lines of L4 L2
  measures "d7" diameter of A0
  measures "d8" diameter of A1
extrude "押し出し2" add sketch "スケッチ5" along normal blind 3 contours L3 L5 L1 L16 | L3 L4 A1 L5 | L5 A1 L4 L1 | L3 L2 L1 L4 | A1
extrude "押し出し3" cut sketch "スケッチ5" along normal mid plane 20 contours A0 | A1
extrude "押し出し4" add sketch "スケッチ4" along normal blind 1 contours A18 | A34 L173 | L173 A34
mirror "ミラー1" about plane through (0, 0, 0) normal (1, 0, 0) of "押し出し1", "押し出し2", "押し出し3"
extrude "押し出し6" add sketch "スケッチ4" along normal blind 1 contours A32 | A33
